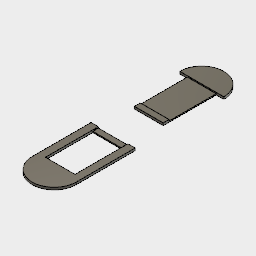
Glued (Autodesk Fusion 360 design; units mm, degrees)
Autodesk Fusion 360 part; units mm, degrees
sketch "Base" plane through (0, 0, 0) normal (0, 1, 0) x (1, 0, 0)
  line L0 (-7.4998, -15.0512) -> (7.5002, -15.0512)
  line L1 (7.5002, -15.0512) -> (7.5002, 4.9488)
  line L2 (7.5002, 4.9488) -> (-7.4998, 4.9488)
  line L3 (-7.4998, 4.9488) -> (-7.4998, -15.0512)
  arc A0 (7.5002, 4.9488) -> (-7.4998, 4.9488) centre (0.0002, 4.9488) ccw
  arc A1 (-7.4998, -15.0512) -> (7.5002, -15.0512) centre (0.0002, -15.0512) ccw
  line L4 (0.0002, -15.0512) -> (-7.4998, -15.0512) construction
  line L5 (0.0002, -15.0512) -> (7.5002, -15.0512) construction
  line L6 (-5, 3) -> (5, 3)
  line L7 (5, 3) -> (5, -13)
  line L8 (5, -13) -> (-5, -13)
  line L9 (-5, -13) -> (-5, 3)
  line L10 (-5, 3) -> (5, 3)
  line L11 (5, 3) -> (5, 4.9488)
  line L12 (5, 4.9488) -> (-5, 4.9488)
  line L13 (-5, 4.9488) -> (-5, 3)
  line L14 (-5, -11) -> (5, -11)
  line L15 (5, -11) -> (5, -13)
  line L16 (5, -13) -> (-5, -13)
  line L17 (-5, -13) -> (-5, -11)
  dimension "d2" = 15
  dimension "d3" = 20
  dimension "d4" = 180
  constraint horizontal L0
  constraint vertical L1
  constraint horizontal L2
  constraint vertical L3
  constraint midpoint L2
  constraint midpoint L0 origin
  constraint horizontal L6
  constraint vertical L7
  constraint horizontal L8
  constraint vertical L9
  constraint horizontal L10
  constraint vertical L11
  constraint horizontal L12
  constraint vertical L13
  constraint coincident L2
  constraint horizontal L14
  constraint vertical L15
  constraint horizontal L16
  constraint vertical L17
  constraint coincident L9 origin
  measures "d3" distance of origin
  measures "d4" angle of L4 L5
extrude "Extrude1" add sketch "Base" along normal blind 0.8 contours L0 L1 L2 L3 L7 L8 L9 L11 L13 L15 L16 L17 | L0 A1 makes body 1
extrude "Extrude2" add sketch "Base" along normal blind 0.4 contours L2 L6 L10 L11 L12 L13 bodies 1
move_body "MoveBody1" bodies 1 to x (1, 0, 0) y (0, 1, 0) z (0, 0, 1) at (0, 0, 30)
extrude "Extrude3" add sketch "Base" along normal blind 0.8 separate body contours L2 A0 L12 | L7 L8 L9 L14 L15 L16 L17 makes body 2 at (-1.6667, 0, 11.6667) makes body 3 at (-1.42, 0, -10.6388)
extrude "Extrude4" add sketch "Base" along normal blind 0.4 contours L2 L6 L10 L11 L12 L13 | L6 L7 L9 L10 L14 bodies 2 3
move_face "OffsetFaces1" offset -0.1 1 faces at (-5, 0.4, 12.3333) on bodies 2
move_face "OffsetFaces2" offset -0.1 1 faces at (5, 0.4, 12.3333) on bodies 2
sketch "Sketch3" plane through (0, 0, 0) normal (0, 1, 0) x (1, 0, 0)
sketch "Sketch4" plane through (0, 0.4, 0) normal (0, 1, 0) x (-1, 0, 0)
  line L0 (-4.9, 11) -> (-4.9, -4.9488)
  line L1 (-4.9, -4.9488) -> (4.9, -4.9488)
  line L2 (4.9, -4.9488) -> (4.9, 11)
  line L3 (4.9, 11) -> (-4.9, 11)
sketch "Sketch5" plane through (0, 0.8, 0) normal (0, 1, 0) x (-1, 0, 0)
  line L0 (-5, 25.0512) -> (-5, 43)
  line L1 (-5, 43) -> (5, 43)
  line L2 (5, 43) -> (5, 25.0512)
  line L3 (5, 25.0512) -> (7.4998, 25.0512)
  line L4 (7.4998, 25.0512) -> (7.4998, 45.0512)
  arc A0 (7.4998, 45.0512) -> (-7.5002, 45.0512) centre (-0.0002, 45.0512) ccw
  line L5 (-7.5002, 45.0512) -> (-7.5002, 25.0512)
  line L6 (-7.5002, 25.0512) -> (-5, 25.0512)
  line L7 (5, 44) -> (-5, 44)
  line L8 (-5, 44) -> (-5, 50)
  line L9 (-5, 50) -> (5, 50)
  line L10 (5, 50) -> (5, 44)
  constraint horizontal L7
  constraint vertical L8
  constraint horizontal L9
  constraint vertical L10
